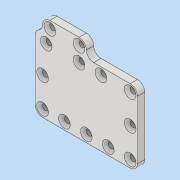
# Autodesk Inventor part: foreElectronicsSealingWallFrontCap
Saved by Autodesk Inventor 2017 (Build 210142000, 142)
## iProperties
Created: 2016-12-09
Part Number: foreElectronicsSealingWallFrontCap
Material: ABS Plastic
Document SubType Name: Modeling
Designer: techn
Density: 1.06 g/cm^3
Appearance: Smooth - White
Author: techn
Autodesk Inventor part; units mm, degrees
ref_plane "YZ Plane" through (0, 0, 0) normal (1, 0, 0) x (0, 1, 0)
ref_plane "XZ Plane" through (0, 0, 0) normal (0, 1, 0) x (-1, 0, 0)
ref_plane "XY Plane" through (0, 0, 0) normal (0, 0, 1) x (1, 0, 0)
sketch "Sketch4" plane through (0, 0, 0) normal (0, 0, 1) x (1, 0, 0)
  line L0 (15.875, 9.525) -> (15.875, -9.525)
  line L1 (15.875, -9.525) -> (-15.875, -9.525)
  line L2 (-15.875, -9.525) -> (-15.875, 9.525)
  line L3 (-15.875, 9.525) -> (-12.7, 9.525)
  line L4 (-12.7, 9.525) -> (-12.7, 15.875)
  line L5 (-12.7, 15.875) -> (-6.35, 15.875)
  line L6 (-6.35, 15.875) -> (-6.35, 9.525)
  line L7 (-6.35, 9.525) -> (15.875, 9.525)
  line L8 (0, 22.225) -> (-19.05, 22.225)
  line L9 (-19.05, 22.225) -> (-19.05, 15.875)
  line L10 (-19.05, 15.875) -> (-22.225, 15.875)
  line L11 (-22.225, 15.875) -> (-22.225, -15.875)
  line L12 (-22.225, -15.875) -> (22.225, -15.875)
  line L13 (22.225, -15.875) -> (22.225, 15.875)
  line L14 (22.225, 15.875) -> (0, 15.875)
  line L15 (0, 15.875) -> (0, 22.225)
  circle A0 centre (-15.875, 19.05) radius 1.27
  circle A1 centre (-3.175, 19.05) radius 1.27
  circle A2 centre (-3.175, 12.7) radius 1.27
  circle A3 centre (6.35, 12.7) radius 1.27
  circle A4 centre (19.05, 12.7) radius 1.27
  circle A5 centre (19.05, 0) radius 1.27
  circle A6 centre (19.05, -12.7) radius 1.27
  circle A7 centre (-19.05, 0) radius 1.27
  circle A8 centre (-19.05, -12.7) radius 1.27
  circle A9 centre (-9.525, -12.7) radius 1.27
  circle A10 centre (0, -12.7) radius 1.27
  circle A11 centre (9.525, -12.7) radius 1.27
  circle A12 centre (-17.4625, 12.7) radius 1.27
  point P0 (0, 0)
  point P1 (0, 0)
  dimension "d64" = 2.54
  dimension "d65" = 2.54
  dimension "d66" = 2.54
  dimension "d67" = 2.54
  dimension "d68" = 2.54
  dimension "d69" = 2.54
  dimension "d70" = 2.54
  dimension "d71" = 2.54
  dimension "d72" = 2.54
  dimension "d73" = 2.54
  dimension "d74" = 2.54
  dimension "d75" = 2.54
  dimension "d76" = 3.175
  dimension "d77" = 3.175
  dimension "d78" = 3.175
  dimension "d79" = 3.175
  dimension "d80" = 3.175
  dimension "d81" = 3.175
  dimension "d82" = 9.525
  dimension "d83" = 9.525
  dimension "d84" = 9.525
  dimension "d85" = 9.525
  dimension "d86" = 2.54
  dimension "d87" = 4.7625
  dimension "d88" = 3.175
  constraints: 32 end point, 13 centre point, 8 horizontal alignment, 4 vertical alignment
  measures "d64" diameter of A0
  measures "d65" diameter of A1
  measures "d66" diameter of A2
  measures "d67" diameter of A3
  measures "d68" diameter of A4
  measures "d69" diameter of A5
  measures "d70" diameter of A6
  measures "d71" diameter of A7
  measures "d72" diameter of A8
  measures "d73" diameter of A9
  measures "d74" diameter of A10
  measures "d75" diameter of A11
  measures "d76" distance from line of A0.centre L9
  measures "d77" distance from line of L8 A0.centre
  measures "d78" distance from line of L15 A2.centre
  measures "d79" distance from line of L11 A8.centre
  measures "d80" distance from line of L12 A8.centre
  measures "d81" distance from line of A4.centre L0
  measures "d82" distance of A3.centre A2.centre
  measures "d83" distance of A6.centre A11.centre
  measures "d84" distance of A10.centre A11.centre
  measures "d85" distance of A9.centre A10.centre
  measures "d86" diameter of A12
  measures "d87" distance from line of A12.centre L11
  measures "d88" distance from line of L10 A12.centre
extrude "Extrusion3" add sketch "Sketch4" along normal blind 3.175 contours L0 L1 L2 L3 L4 L5 L6 L7 | L15 L14 L13 L12 L11 L10 L9 L8
chamfer "Chamfer3" distance 1.27 angle 45 13 edges at (-17.145, 19.05, 3.175) (-4.445, 19.05, 3.175) (-4.445, 12.7, 3.175) (5.08, 12.7, 3.175) (17.78, 12.7, 3.175) (17.78, 0, 3.175) (17.78, -12.7, 3.175) (8.255, -12.7, 3.175) (-1.27, -12.7, 3.175) (-10.795, -12.7, 3.175) (-20.32, -12.7, 3.175) (-20.32, 0, 3.175) (-18.7325, 12.7, 3.175)
fillet "Fillet2" radius 3.175 8 edges at (22.225, 15.875, 1.5875) (0, 15.875, 1.5875) (0, 22.225, 1.5875) (-19.05, 22.225, 1.5875) (-19.05, 15.875, 1.5875) (-22.225, 15.875, 1.5875) (-22.225, -15.875, 1.5875) (22.225, -15.875, 1.5875)
equation "\"d84\" = d83"
equation "\"d85\" = d83"
body "Solid3"
